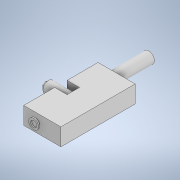
# Autodesk Inventor part: vacuumGenerator
Saved by Autodesk Inventor 2021 (Build 250183000, 183)
## iProperties
Created: 2021-01-06
Part Number: vacuumGenerator
Material: Generic
Document SubType Name: Modeling
Designer: awitc
Density: 1 g/cm^3
Appearance: Default
Author: awitc
Autodesk Inventor part; units mm, degrees
ref_plane "YZ Plane" through (0, 0, 0) normal (1, 0, 0) x (0, 1, 0)
ref_plane "XZ Plane" through (0, 0, 0) normal (0, 1, 0) x (-1, 0, 0)
ref_plane "XY Plane" through (0, 0, 0) normal (0, 0, 1) x (1, 0, 0)
sketch "Sketch1" plane through (0, 0, 0) normal (0, 1, 0) x (-1, 0, 0)
  line L0 (0, 0) -> (30, 0)
  line L1 (30, 0) -> (30, -60)
  line L2 (30, -60) -> (0, -60)
  line L3 (0, -60) -> (0, 0)
  dimension "d0" = 30
  dimension "d1" = 60
  constraints: 8 end point, 2 parallel, 1 horizontal, 1 perpendicular
  measures "d0" distance of L1.end L2.end
  measures "d1" distance of L0.end L1.end
extrude "Extrusion1" add sketch "Sketch1" along normal blind 14
sketch "Sketch2" plane through (-30, 0, 0) normal (0, 0, 1) x (1, 0, 0)
  line L0 (0, 0) -> (0, 14) projected
  line L1 (0, 7) -> (10, 7)
  circle A0 centre (10, 7) radius 3
  point P0 (30, 0)
  dimension "d4" = 10
  dimension "d5" = 6
  constraints: 2 end point, 1 centre point, 1 coincident, 1 horizontal, 1 midpoint
  measures "d4" distance of L1.start L1.end
  measures "d5" diameter of A0
extrude "Extrusion2" add sketch "Sketch2" along normal blind 1
sketch "Sketch3" plane through (-20, 7, 1) normal (0, 0, 1) x (1, 0, 0)
  circle A0 centre (0, 0) radius 4
  point P0 (20, -7)
  dimension "d8" = 8
  constraints: 1 centre point
  measures "d8" diameter of A0
extrude "Extrusion3" add sketch "Sketch3" along normal blind 1
sketch "Sketch4" plane through (-20, 7, 2) normal (0, 0, 1) x (1, 0, 0)
  circle A0 centre (0, 0) radius 2.5
  point P0 (20, -7)
  dimension "d11" = 5
  constraints: 1 centre point
  measures "d11" diameter of A0
extrude "Extrusion4" cut sketch "Sketch4" against normal blind 1
sketch "Sketch5" plane through (0, 0, -60) normal (0, 0, -1) x (-1, 0, 0)
  line L0 (30, 0) -> (30, 14) projected
  line L1 (30, 7) -> (20, 7)
  circle A0 centre (20, 7) radius 3
  point P0 (0, 0)
  dimension "d14" = 10
  dimension "d15" = 6
  constraints: 2 end point, 1 centre point, 1 coincident, 1 horizontal, 1 midpoint
  measures "d14" distance of L1.start L1.end
  measures "d15" diameter of A0
extrude "Extrusion5" add sketch "Sketch5" along normal blind 1
sketch "Sketch6" plane through (-20, 7, -61) normal (0, 0, -1) x (-1, 0, 0)
  circle A0 centre (0, 0) radius 4.5
  point P0 (-20, -7)
  dimension "d18" = 9
  constraints: 1 centre point
  measures "d18" diameter of A0
extrude "Extrusion6" add sketch "Sketch6" along normal blind 30
sketch "Sketch7" plane through (-30, 0, -60) normal (-1, 0, 0) x (0, 0, 1)
  line L0 (60, 0) -> (30, 0)
  line L1 (0, 0) -> (60, 0) projected
  line L2 (30, 0) -> (35, 0)
  line L3 (35, 0) -> (35, 14)
  line L4 (0, 14) -> (60, 14) projected
  line L5 (35, 14) -> (25, 14)
  line L6 (25, 14) -> (25, 0)
  line L7 (25, 0) -> (30, 0)
  circle A0 centre (30, 7) radius 4.5
  dimension "d21" = 5
  dimension "d22" = 10
  dimension "d23" = 9
  constraints: 12 end point, 4 perpendicular, 3 point on line, 1 centre point, 1 midpoint
  measures "d21" distance of L0.end L2.end
  measures "d22" distance of L3.end L5.end
  measures "d23" diameter of A0
extrude "Extrusion7" cut sketch "Sketch7" against normal blind 10
sketch "Sketch8" plane through (-30, 7, -30) normal (-1, 0, 0) x (0, 0, 1)
  circle A0 centre (0, 0) radius 4.5
  point P0 (30, -7)
  constraints: 1 centre point
extrude "Extrusion8" add sketch "Sketch8" along normal blind 10
sketch "Sketch9" plane through (-40, 7, -30) normal (-1, 0, 0) x (0, 0, 1)
  circle A0 centre (0, 0) radius 2
  point P0 (30, -7)
  dimension "d28" = 4
  constraints: 1 centre point
  measures "d28" diameter of A0
extrude "Extrusion9" add sketch "Sketch9" along normal blind 1
sketch "Sketch10" plane through (-41, 7, -30) normal (-1, 0, 0) x (0, 0, 1)
  circle A0 centre (0, 0) radius 3
  line L0 (0, -3) -> (-2.5981, -1.5)
  line L1 (-2.5981, -1.5) -> (-2.5981, 1.5)
  line L2 (-2.5981, 1.5) -> (0, 3)
  line L3 (0, 3) -> (2.5981, 1.5)
  line L4 (2.5981, 1.5) -> (2.5981, -1.5)
  line L5 (2.5981, -1.5) -> (0, -3)
  point P0 (30, -7)
  dimension "d31" = 6
  constraints: 12 end point, 1 coincident, 1 vertical alignment, 15 other
extrude "Extrusion10" add sketch "Sketch10" along normal blind 1 contours L4 L5 L0 L1 L2 L3
sketch "Sketch11" plane through (-20, 7, -91) normal (0, 0, -1) x (-1, 0, 0)
  line L0 (0, -4.5) -> (0, 4.5) projected
  circle A0 centre (0, 0) radius 2.5
  point P0 (-20, -7)
  dimension "d34" = 5
  constraints: 1 centre point, 1 midpoint
  measures "d34" diameter of A0
extrude "Extrusion11" cut sketch "Sketch11" against normal blind 10
body "Solid1"
